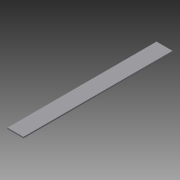
# Autodesk Inventor part: 14in Steel beam
Saved by Autodesk Inventor 2015 (Build 190159000, 159)
## iProperties
Created: 2017-01-05
Part Number: 14in Steel beam
Material: Generic
Document SubType Name: Modeling
Designer: ps2du
Density: 1 g/cm^3
Appearance: Default
Author: ps2du
Autodesk Inventor part; units mm, degrees
ref_plane "YZ Plane" through (0, 0, 0) normal (1, 0, 0) x (0, 1, 0)
ref_plane "XZ Plane" through (0, 0, 0) normal (0, 1, 0) x (-1, 0, 0)
ref_plane "XY Plane" through (0, 0, 0) normal (0, 0, 1) x (1, 0, 0)
sketch "Sketch1" plane through (0, 0, 0) normal (0, 0, 1) x (1, 0, 0)
  line L0 (0, 0) -> (38.1, 0)
  line L1 (38.1, 0) -> (38.1, 3.175)
  line L2 (38.1, 3.175) -> (0, 3.175)
  line L3 (0, 3.175) -> (0, 0)
  dimension "d0" = 38.1
  dimension "d1" = 3.175
  constraints: 8 end point, 2 parallel, 1 horizontal, 1 perpendicular
  measures "d0" distance of L2.end L1.end
  measures "d1" distance between parallel lines of L0 L2
extrude "Extrusion1" add sketch "Sketch1" along normal blind 355.6
body "Solid1"
